Autodesk Inventor part; units mm, degrees
(part 2 of 2)
  arc A230 (22.2555, -40.324) -> (22.3762, -39.8361) centre (13, -37.7752) ccw construction
  arc A231 (20.8284, -40.3788) -> (22.2555, -40.324) centre (21.313, -34.3954) ccw construction
  arc A232 (20.6814, -40.785) -> (20.8284, -40.3788) centre (13, -37.7752) ccw construction
  arc A233 (21.7428, -41.7405) -> (20.6814, -40.785) centre (17.2242, -45.6926) ccw construction
  arc A234 (21.5233, -42.1926) -> (21.7428, -41.7405) centre (13, -37.7752) ccw construction
  arc A235 (20.116, -41.9495) -> (21.5233, -42.1926) centre (21.8341, -36.1976) ccw construction
  arc A236 (19.8878, -42.3162) -> (20.116, -41.9495) centre (13, -37.7752) ccw construction
  arc A237 (20.7273, -43.4715) -> (19.8878, -42.3162) centre (15.4858, -46.3978) ccw construction
  arc A238 (20.4186, -43.8681) -> (20.7273, -43.4715) centre (13, -37.7752) ccw construction
  arc A239 (19.0926, -43.3378) -> (20.4186, -43.8681) centre (21.969, -38.0688) ccw construction
  arc A240 (18.7931, -43.649) -> (19.0926, -43.3378) centre (13, -37.7752) ccw construction
  circle A241 centre (14.5, -58.0698) radius 5 projected
  circle A242 centre (13, -37.7752) radius 9.6 construction
  circle A243 centre (8.9947, -49.7216) radius 8 construction
  circle A244 centre (8.9947, -49.7216) radius 8.4
  circle A245 centre (13, -37.7752) radius 10
  point P0 (16.9144, -48.5908)
  point P1 (16.9313, -46.97)
  point P2 (16.5028, -53.4884)
  point P3 (9.5001, -58.1064)
  point P4 (4.3207, -42.7421)
  dimension "d21" = 0.4
  dimension "d22" = 0.4
  constraints: 8 end point, 2 centre point, 2 coincident, 2 parallel, 1 horizontal, 1 perpendicular, 1 point on circle, 6 other
extrude "Extrusion7" add sketch "Sketch3" against normal blind 4.5
sketch "Sketch4" plane through (0, -2.774, -8.5) normal (0, 0, -1) x (-1, 0, 0)
  line L0 (1.5, 3.274) -> (1.5, 19.274) projected
  line L1 (2.5, 3.274) -> (1.5, 3.274) projected
  line L2 (2.5, 19.274) -> (2.5, 3.274) projected
  line L3 (2.5, 19.274) -> (1.5, 19.274) projected
  line L4 (2.5, 19.274) -> (2.5, 19.774)
  line L5 (2.5, 19.774) -> (1, 19.774)
  line L6 (1, 19.774) -> (1, 3.274)
  line L7 (23.2, 2.774) -> (0, 2.774) projected
  line L8 (1, 3.274) -> (1.5, 3.274)
  dimension "d27" = 0.5
  dimension "d28" = 0.5
  constraints: 8 end point, 2 perpendicular, 1 collinear, 1 vertical
  measures "d27" distance between parallel lines of L5 L3
  measures "d28" distance between parallel lines of L6 L0
extrude "Extrusion8" cut sketch "Sketch4" against normal blind 7.5
sketch "Sketch5" plane through (0, -2.774, -8.5) normal (0, 0, -1) x (-1, 0, 0)
  line L0 (1.5, 3.274) -> (1.5, 19.274) projected
  line L1 (2.5, 3.274) -> (1.5, 3.274) projected
  line L2 (2.5, 19.274) -> (2.5, 3.274) projected
  line L3 (2.5, 19.274) -> (1.5, 19.274) projected
  line L4 (2.5, 19.274) -> (2.5, 20.774)
  line L5 (2.5, 20.774) -> (0, 20.774)
  line L6 (0, 2.774) -> (0, 68.0698) projected
  line L7 (0, 2.774) -> (0, 20.774)
  line L8 (0, 2.774) -> (2.5, 2.774)
  line L9 (2.5, 2.774) -> (2.5, 3.274)
  line L10 (1, 19.774) -> (1, 2.774)
  line L11 (1, 2.774) -> (3, 2.774)
  line L12 (3, 2.774) -> (3, 19.774)
  line L13 (3, 19.774) -> (1, 19.774)
  line L14 (1.5, 16.174) -> (1.5, 12.674) projected
  line L15 (1.5, 16.174) -> (0, 16.174) projected
  line L16 (0, 12.674) -> (0, 16.174) projected
  line L17 (1.5, 12.674) -> (0, 12.674) projected
  line L18 (1.5, 9.874) -> (1.5, 6.374) projected
  line L19 (1.5, 9.874) -> (0, 9.874) projected
  line L20 (0, 6.374) -> (0, 9.874) projected
  line L21 (1.5, 6.374) -> (0, 6.374) projected
  line L22 (-0.5, 16.674) -> (2, 16.674)
  line L23 (2, 16.674) -> (2, 12.174)
  line L24 (2, 12.174) -> (-0.5, 12.174)
  line L25 (-0.5, 12.174) -> (-0.5, 16.674)
  line L26 (-0.5, 10.374) -> (2, 10.374)
  line L27 (2, 10.374) -> (2, 5.874)
  line L28 (2, 5.874) -> (-0.5, 5.874)
  line L29 (-0.5, 5.874) -> (-0.5, 10.374)
  line L30 (2.5, 3.274) -> (1, 3.274) projected
  line L31 (1.5, 3.274) -> (1, 3.274)
  point P0 (0, 16.674)
  point P1 (1, 16.674)
  point P2 (2.5, 19.774)
  point P3 (0, 10.374)
  point P4 (1, 10.374)
  point P5 (1, 12.174)
  point P6 (0, 12.174)
  point P7 (1, 5.874)
  point P8 (0, 5.874)
  dimension "d31" = 0.5
  dimension "d32" = 1
  dimension "d33" = 0.5
  dimension "d34" = 0.5
  constraints: 36 end point, 3 perpendicular, 2 collinear, 2 point on line, 1 vertical, 9 other
  measures "d31" distance between parallel lines of L0 L10
  measures "d32" distance between parallel lines of L5 L13
  measures "d33" distance between parallel lines of L15 L22
  measures "d34" distance between parallel lines of L19 L26
ref_plane "Work Plane6" through (-2.5, 0.5, -17) normal (0, 0, -1) x (0, 1, 0)
extrude "Extrusion9" add sketch "Sketch5" along normal blind 8 contours L1 L9 L8 L10 L30 | L10 L8 L6 L28 | L26 L6 L24 L10 | L13 L10 L22 L6 L5 L4
sketch "Sketch7" plane through (0, -2.774, -8.5) normal (0, 0, -1) x (-1, 0, 0)
  circle A0 centre (20.6284, 52.9275) radius 2.25 projected
  circle A1 centre (8.3716, 63.2121) radius 2.25 projected
  point P0 (0, 2.774)
extrude "Extrusion10" cut sketch "Sketch7" against normal blind 2.6
sketch "Sketch8" plane through (-8.3716, 60.4381, -5.9) normal (0, 0, -1) x (-1, 0, 0)
  circle A0 centre (0, 0) radius 1.0564 projected
  circle A1 centre (12.2567, -10.2846) radius 1.0564 projected
  circle A2 centre (6.1284, -5.1423) radius 5 projected
  circle A3 centre (6.1284, -5.1423) radius 13.85 projected
  point P0 (-8.3716, -60.4381)
hole "Hole2" at (-20.6284, 50.1535, -5.9) at (-8.3716, 60.4381, -5.9) direction (0, 0, 1) diameter 2.5 depth 8.8 counterbore diameter 4.5 counterbore depth 2.5
sketch "Sketch6" plane through (-23.2, 65.2958, 0.6) normal (0, 1, 0) x (1, 0, 0)
  line L0 (0, 9.1) -> (0, 0) projected
  line L1 (23.2, 0) -> (0, 0) projected
  line L2 (0, 9.1) -> (23.2, 9.1) projected
  line L3 (0, 4.55) -> (23.2, 4.55)
  line L4 (0.2, 9.1) -> (20.2, 9.1) projected
  line L5 (17.2, 9.1) -> (17.2, 0)
  circle A0 centre (10.7, 4.55) radius 3.5
  circle A1 centre (3.5, 4.55) radius 3.5
  line L6 (23.2, 9.1) -> (23.2, 0) projected
  point P0 (23.2, 0.6)
  point P1 (11.6, 4.55)
  point P2 (19.8, 4.55)
  point P3 (6.2687, 9.1)
  point P4 (18.8793, 9.1)
  dimension "d52" = 7
  dimension "d53" = 7
  dimension "d55" = 0
  dimension "d67" = 3
  dimension "d102" = 6
  constraints: 5 point on line, 4 end point, 3 midpoint, 2 centre point, 1 perpendicular
  measures "d52" diameter of A1
  measures "d53" diameter of A0
  measures "d55" distance edge to line of A1 L0
  measures "d67" distance edge to line of A0 L5
  measures "d102" distance between parallel lines of L6 L5
hole "Hole1" at (-19.7, 65.2958, -3.95) at (-12.5, 65.2958, -3.95) direction (0, -1, 0) diameter 4 depth 4 counterbore diameter 4.5 counterbore depth 0.5
sketch "Sketch9" plane through (0, 0, -1.1) normal (0, 0, -1) x (-1, 0, 0)
  arc A0 (9.5001, 55.3324) -> (4.3207, 39.9681) centre (8.9947, 46.9477) ccw projected
  point P0 (0, 0)
hole "Hole3" at (-8.9947, 46.9477, -1.1) direction (0, 0, 1) diameter 2.5 depth 1.5
sketch "Sketch10" plane through (0, -2.774, -8.5) normal (0, 0, -1) x (-1, 0, 0)
  circle A0 centre (20.6284, 52.9275) radius 2.25 projected
  circle A1 centre (8.3716, 63.2121) radius 2.25 projected
  line L0 (2.5, 20.774) -> (2.5, 19.774) projected
  line L1 (2.5, 19.774) -> (2.5, 3.274) projected
  line L2 (2.5, 3.274) -> (2.5, 2.774) projected
  line L3 (2.5, 2.774) -> (23.2, 2.774) projected
  line L4 (23.2, 2.774) -> (23.2, 68.0698) projected
  line L5 (23.2, 68.0698) -> (0, 68.0698) projected
  line L6 (0, 68.0698) -> (0, 20.774) projected
  line L7 (0, 20.774) -> (2.5, 20.774) projected
  arc A2 (4.3207, 42.7421) -> (16.9313, 46.97) centre (13, 37.7752) ccw projected
  arc A3 (9.5001, 58.1064) -> (4.3207, 42.7421) centre (8.9947, 49.7216) ccw projected
  arc A4 (16.5028, 53.4884) -> (9.5001, 58.1064) centre (14.5, 58.0698) ccw projected
  arc A5 (16.9313, 46.97) -> (16.5028, 53.4884) centre (8.9947, 49.7216) ccw projected
  line L8 (23.2, 7.524) -> (0, 7.524)
  line L9 (0, 2.774) -> (0, 68.0698) projected
  line L10 (0, 15.774) -> (23.2, 15.774)
  line L11 (23.2, 21.774) -> (0, 21.774)
  circle A6 centre (3.5, 64.5698) radius 3.5
  circle A7 centre (3.5, 64.5698) radius 2.5
  line L12 (23.2, 68.0698) -> (0, 68.0698) projected
  line L13 (0, 68.0698) -> (0, 20.774) projected
  circle A8 centre (19.7877, 48.2613) radius 3.5
  circle A9 centre (20.6284, 52.9275) radius 2.25 projected
  circle A10 centre (19.7877, 48.2613) radius 2.5
  circle A11 centre (3.5, 28.1835) radius 3.5
  circle A12 centre (19.7, 25.274) radius 3.5
  line L14 (23.2, 2.774) -> (23.2, 68.0698) projected
  circle A13 centre (7, 11.649) radius 3.5
  circle A14 centre (19.2, 11.649) radius 3.5
  point P0 (23.2, 52.8075)
  point P1 (23.2, 54.1548)
  dimension "d76" = 4.75
  dimension "d77" = 8.25
  dimension "d78" = 6
  dimension "d79" = 7
  dimension "d80" = 5
  dimension "d81" = 7
  dimension "d82" = 5
  dimension "d83" = -0.0087
  dimension "d84" = -0.0087
  dimension "d85" = -0.0087
  dimension "d86" = 7
  dimension "d87" = 7
  dimension "d88" = 7
  dimension "d89" = 7
  dimension "d90" = 4.125
  dimension "d91" = 4.125
  dimension "d92" = 7
  dimension "d93" = 4
  dimension "d94" = 4.125
  constraints: 8 centre point, 6 end point, 6 point on line, 6 tangent, 2 coincident, 2 perpendicular, 1 horizontal, 1 other
  measures "d76" distance between parallel lines of L8 L3
  measures "d77" distance between parallel lines of L10 L8
  measures "d78" distance between parallel lines of L10 L11
  measures "d79" diameter of A6
  measures "d80" diameter of A7
  measures "d81" diameter of A8
  measures "d82" diameter of A10
  measures "d86" diameter of A11
  measures "d87" diameter of A12
  measures "d88" diameter of A13
  measures "d89" distance from line of L9 A13.centre
  measures "d90" distance from line of L10 A13.centre
  measures "d91" distance from line of L8 A13.centre
  measures "d92" diameter of A14
  measures "d93" distance from line of L14 A14.centre
  measures "d94" distance from line of L10 A14.centre
hole "Hole4" at (-3.5, 61.7958, -8.5) at (-19.7877, 45.4874, -8.5) at (-19.7, 22.5, -8.5) at (-3.5, 25.4095, -8.5) at (-7, 8.875, -8.5) at (-19.2, 8.875, -8.5) direction (0, 0, 1) diameter 4 depth 4 counterbore diameter 4.5 counterbore depth 0.5
sketch "Sketch11" plane through (-23.2, 25.2765, 0.6) normal (-1, 0, 0) x (0, 0, 1)
  circle A0 centre (-6.4, -22.5765) radius 2.7
  line L0 (-9.1, -25.2765) -> (-9.1, 40.0194) projected
  line L1 (-9.1, -25.2765) -> (0, -25.2765) projected
  line L2 (-4.6, -15.7765) -> (-4.6, -5.7765) projected
  line L3 (-0.6, -5.7765) -> (-0.6, -15.7765) projected
  line L4 (-0.6, -16.5483) -> (-4.6, -16.5483) projected
  line L5 (-0.6, -6.7398) -> (-0.6, -16.5483) projected
  line L6 (-0.6, -12.3483) -> (-9.1, -12.3483)
  line L7 (-9.1, 27.1271) -> (-4, 27.1271) projected
  line L8 (-4, 27.1271) -> (-4, 22.6271) projected
  line L9 (-9.1, 22.6271) -> (-9.1, 27.1271) projected
  line L10 (-9.1, 27.1271) -> (0, 27.1271)
  line L11 (0, 40.0194) -> (0, 0) projected
  circle A1 centre (-3, 30.1271) radius 3
  line L12 (-8.6, 22.2109) -> (-8.6, 18.2109) projected
  line L13 (-5.1, 22.2109) -> (-5.1, 18.2109) projected
  line L14 (-9.1, 18.2109) -> (0, 18.2109)
  circle A2 centre (-3, 20.2109) radius 3
  line L15 (-8.6, -0.7765) -> (-8.6, -4.7765) projected
  line L16 (-5.1, -0.7765) -> (-5.1, -4.7765) projected
  line L17 (-9.1, 40.0194) -> (-9.1, -7.2765) projected
  line L18 (-9.1, -0.7765) -> (-0.6, -0.7765)
  line L19 (-0.6, 0) -> (-0.6, -1.801) projected
  point P0 (-0.6, -25.2765)
  point P1 (-4.6, -20.5641)
  point P2 (-4.85, -12.3483)
  dimension "d103" = 5.3999
  dimension "d104" = 4.2
  dimension "d105" = 4.25
  dimension "d106" = 4.25
  dimension "d107" = 6
  dimension "d109" = 6.1
  dimension "d110" = 6
  dimension "d113" = 2
  constraints: 9 point on line, 8 end point, 3 horizontal, 3 tangent, 2 centre point, 2 perpendicular, 1 midpoint, 1 vertical, 3 other
  measures "d104" distance between parallel lines of L6 L4
  measures "d105" distance from line of point (-4.85, -12.348) L0
  measures "d106" distance from line of L3 point (-4.85, -12.348)
  measures "d107" diameter of A1
  measures "d109" distance from line of L0 A1.centre
  measures "d110" diameter of A2
  measures "d113" distance from line of A2.centre L14
hole "Hole5" at (-23.2, 12.9282, -4.25) at (-23.2, 45.4874, -2.4) at (-23.2, 55.4035, -2.4) at (-23.2, 2.7, -5.8) direction (1, 0, 0) diameter 4 depth 3.5 counterbore diameter 4.5 counterbore depth 0.5
body "Solid3"
